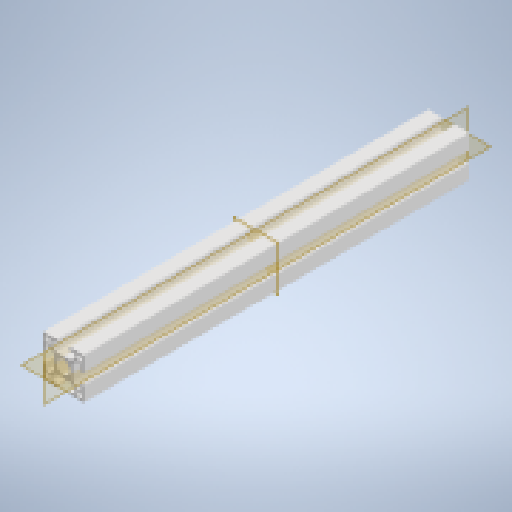
# Autodesk Inventor part: perfil_30x30_003
Saved by Autodesk Inventor 2026 (Build 300175000, 175)
## iProperties
Created: 2025-11-25
Part Number: perfil_30x30_003
Material: Generic
Document SubType Name: Modeling
Designer: Carlos Dias
Density: 1 g/cm^3
Appearance: Default
Author: Carlos Dias
Autodesk Inventor part; units mm, degrees
sketch "Sketch1" plane through (0, 0, 0) normal (0, 0, 1) x (1, 0, 0)
  circle A0 centre (0, 0) radius 5
  line L0 (-15, 15) -> (0, 15) construction
  line L1 (-15, 15) -> (-15, 0) construction
  line L2 (-15, 15) -> (0, 0) construction
  circle A1 centre (-11.5, 11.5) radius 2.25
  line L3 (-15, 15) -> (-4.1, 15)
  line L4 (-5.5858, 7) -> (0, 7)
  line L5 (-8.3858, 9.8) -> (-5.5858, 7)
  line L6 (-8.3858, 12.8) -> (-4.1, 12.8)
  line L7 (-4.1, 12.8) -> (-4.1, 14.5)
  line L8 (-4.1, 14.5) -> (-4.6, 14.5)
  line L9 (-4.6, 15) -> (-4.6, 14.5)
  line L10 (-8.3858, 12.8) -> (-8.3858, 9.8)
  line L11 (-15, 15) -> (-15, 4.1)
  line L12 (-15, 4.1) -> (-14.5, 4.1)
  line L13 (-14.5, 4.1) -> (-14.5, 3.6)
  line L14 (-14.5, 3.6) -> (-12.8, 3.6)
  line L15 (-12.8, 3.6) -> (-12.8, 8.3858)
  line L16 (-7, 5.5858) -> (-7, 0)
  line L17 (-9.8, 8.3858) -> (-7, 5.5858)
  line L18 (-12.8, 8.3858) -> (-9.8, 8.3858)
  line L19 (-7, 0) -> (-5, 0)
  line L20 (0, 7) -> (0, 5)
  dimension "d0" = 10
  dimension "d1" = 15
  dimension "d2" = 15
  dimension "d3" = 4.5
  dimension "d4" = 11.5
  dimension "d5" = 4.1
  dimension "d6" = 8
  dimension "d7" = 1
  dimension "d8" = 2.2
  dimension "d9" = 0.5
  dimension "d12" = 3
  constraints: 42 end point, 7 equal length, 7 vertical, 6 horizontal, 5 perpendicular, 4 coincident, 3 vertical alignment, 2 centre point, 2 horizontal alignment, 2 point on circle, 2 point on line, 1 parallel, 1 other
  measures "d0" diameter of A0
  measures "d1" distance of L0.end point (0, 0)
  measures "d2" distance of L0.start L0.end
  measures "d3" diameter of A1
  measures "d4" horizontal distance of point (0, 0) A1.centre
  measures "d5" distance of L0.end L3.end
  measures "d6" distance between parallel lines of L0 L4
  measures "d7" distance between parallel lines of L5 L2
  measures "d8" distance between parallel lines of L0 L6
  measures "d9" distance of L7.end L8.end
  measures "d12" distance of L6.start L5.start
extrude "Extrusion1" add sketch "Sketch1" along normal mid plane 280 contours A0 L19 L16 L17 L18 L15 L14 L13 L12 L11 L3 L9 L8 L7 L6 L10 L5 L4 L20
fillet "Fillet1" radius 0.5 7 edges at (-15, 15, 0) (-8.3858, 12.8, 0) (-8.3858, 9.8, 0) (-5.5858, 7, 0) (-12.8, 8.3858, 0) (-9.8, 8.3858, 0) (-7, 5.5858, 0)
mirror "Mirror1" about plane through (0, 0, 0) normal (1, 0, 0) of "Extrusion1", "Fillet1"
mirror "Mirror2" about plane through (0, 0, 0) normal (0, 1, 0) of "Extrusion1", "Fillet1", "Mirror1"
body "Solid1"
